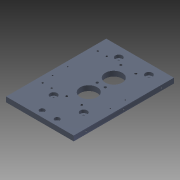
# Autodesk Inventor part: 13_0204_028
Saved by Autodesk Inventor 2012 SP1 (Build 160190100, 190)
## iProperties
Created: 2013-03-27
Part Number: 13_0204_028
Material: Default
Document SubType Name: Modeling
Designer: vogel
Density: 1 g/cm^3
Author: vogel
Autodesk Inventor part; units mm, degrees
ref_plane "YZ Plane" through (0, 0, 0) normal (1, 0, 0) x (0, 1, 0)
ref_plane "XZ Plane" through (0, 0, 0) normal (0, 1, 0) x (-1, 0, 0)
sketch "Skizze1" plane through (0, 0, 0) normal (0, 0, 1) x (1, 0, 0)
  line L0 (-60, 110) -> (60, 110)
  line L1 (60, 110) -> (60, -50)
  line L2 (60, -50) -> (-60, -50)
  line L3 (-60, -50) -> (-60, 110)
  line L4 (-1104, 0) -> (254, 0) projected
  line L5 (0, -83) -> (0, 148) projected
  circle A0 centre (-30, 0) radius 2.7
  circle A1 centre (30, 0) radius 2.7
  line L6 (-910, 115) -> (-40, 115) projected
  point P0 (0, 0)
  dimension "d0" = 110
  dimension "d1" = 120
  dimension "d2" = 60
  dimension "d3" = 5.4
  dimension "d7" = 50
  constraints: 8 end point, 2 centre point, 2 coincident, 2 parallel, 2 point on line, 1 equal radius, 1 horizontal, 1 perpendicular, 1 symmetric about line, 1 other
  measures "d0" distance between parallel lines of L0 L4
  measures "d1" distance of L0.start L0.end
  measures "d2" distance of point (30, 0) point (-30, 0)
  measures "d3" diameter of A0
  measures "d7" distance between parallel lines of L2 L4
extrude "Extrusion1" add sketch "Skizze1" along normal blind 10 contours L0 L5 L4 A0 L3 | L0 L1 L4 A1 L5 | L4 A0 L5 L2 L3 | L4 A1 L1 L2 L5
sketch "Skizze2" plane through (0, 0, 10) normal (0, 0, 1) x (1, 0, 0)
  line L0 (-60, 110) -> (60, 110) projected
  line L1 (0, -82) -> (0, 142) projected
  point P0 (0, 0)
  point P1 (0, 90)
  point P2 (0, 40)
  dimension "d17" = 20
  dimension "d18" = 50
  constraints: 2 point on line
  measures "d17" distance from line of L0 point (0, 90)
  measures "d18" distance of point (0, 90) point (0, 40)
hole "Bohrung2" at (0, 90, 10) at (0, 40, 10) direction (0, 0, -1) diameter 34 end through all
sketch "Skizze5" plane through (0, 0, 10) normal (0, 0, 1) x (1, 0, 0)
  circle A0 centre (30, 0) radius 2.7 projected
  circle A1 centre (-30, 0) radius 2.7 projected
  circle A2 centre (-30, 0) radius 7
  circle A3 centre (30, 0) radius 7
  point P0 (0, 0)
  dimension "d33" = 14
  constraints: 2 centre point, 2 coincident, 1 equal radius
  measures "d33" diameter of A2
extrude "Extrusion2" cut sketch "Skizze5" against normal blind 6
sketch "Skizze6" plane through (-60, 110, 0) normal (0, 1, 0) x (1, 0, 0)
  line L0 (0, -10) -> (120, -10) projected
  line L1 (120, 0) -> (120, -10) projected
  line L2 (0, 0) -> (120, 0) projected
  line L3 (0, 0) -> (0, -10) projected
  point P0 (60, 0)
extrude "Extrusion3" add sketch "Skizze6" along normal blind 40
pattern_linear "Rechteckige Anordnung1" count 2 spacing 130 along (0, 1, 0) of "Extrusion2"
sketch "Skizze8" plane through (0, 0, 10) normal (0, 0, 1) x (1, 0, 0)
  circle A0 centre (30, 130) radius 7 projected
  circle A1 centre (-30, 130) radius 7 projected
  point P0 (0, 0)
  constraints: 2 coincident
hole "Bohrung4" at (-30, 130, 10) at (30, 130, 10) direction (0, 0, -1) diameter 5.4 end through all
sketch "Skizze9" plane through (-60, -50, 0) normal (-1, 0, 0) x (0, 0, 1)
  line L0 (10, 0) -> (10, 200) projected
  line L1 (10, 200) -> (0, 200) projected
  line L2 (0, 0) -> (0, 200) projected
  line L3 (0, 0) -> (10, 0) projected
  point P0 (0, 50)
extrude "Extrusion4" add sketch "Skizze9" along normal blind 15
sketch "Skizze10" plane through (0, 0, 10) normal (0, 0, 1) x (1, 0, 0)
  line L0 (60, 150) -> (-75, 150) projected
  line L1 (-75, 150) -> (-75, -50) projected
  line L2 (60, -50) -> (-75, -50) projected
  line L3 (-75, 120) -> (-28.668, 120)
  line L4 (-53, 93.8234) -> (-53, 98.8806)
  line L5 (60, 150) -> (60, -50) projected
  line L6 (-75, 10) -> (-27.5048, 10)
  point P0 (0, 0)
  point P1 (-62, 120)
  point P2 (-44, 120)
  point P3 (-62, 10)
  point P4 (-44, 10)
  dimension "d50" = 30
  dimension "d51" = 22
  dimension "d52" = 18
  dimension "d60" = 140
  dimension "d61" = 18
  constraints: 6 end point, 6 point on line, 2 perpendicular, 2 symmetric about line, 1 parallel
  measures "d50" distance between parallel lines of L0 L3
  measures "d51" distance between parallel lines of L1 L4
  measures "d52" distance of point (-44, 120) point (-62, 120)
  measures "d60" distance between parallel lines of L0 L6
  measures "d61" distance of point (-44, 10) point (-62, 10)
hole "Bohrung6" at (-62, 120, 10) at (-44, 120, 10) at (-62, 10, 10) at (-44, 10, 10) direction (0, 0, -1) diameter 3.242 end through all thread size "M4x0.7" class "6H" standard "ISO Metric profile"
sketch "Skizze11" plane through (0, 0, 10) normal (0, 0, 1) x (1, 0, 0)
  circle A0 centre (7.5, -46) radius 1.621 projected
  circle A1 centre (7.5, -30) radius 1.621 projected
  circle A2 centre (-7.5, -30) radius 1.621 projected
  circle A3 centre (-7.5, -46) radius 1.621 projected
  line L0 (-25, -26) -> (25, -26) projected
  line L1 (-25, -50) -> (-25, -26) projected
  line L2 (25, -50) -> (-25, -50) projected
  line L3 (25, -26) -> (25, -50) projected
  line L4 (-25, -38) -> (25, -38)
  line L5 (-102, 0) -> (87, 0) projected
  line L6 (0, -90) -> (0, 190) projected
  circle A4 centre (15, -38) radius 2.067 projected
  circle A5 centre (-15, -38) radius 2.067 projected
  point P0 (0, 0)
  point P1 (-15, -38)
  point P2 (15, -38)
  dimension "d69" = 30
  constraints: 2 end point, 2 midpoint, 2 point on line, 1 symmetric about line
  measures "d69" distance of point (15, -38) point (-15, -38)
hole "Bohrung7" at (-15, -38, 10) at (15, -38, 10) direction (0, 0, -1) diameter 5.5 end through all counterbore diameter 10 counterbore depth 5.4
sketch "Skizze12" plane through (60, -50, 10) normal (1, 0, 0) x (0, 0, -1)
  line L0 (0, 200) -> (0, 0) projected
  line L1 (10, 0) -> (0, 0) projected
  line L2 (10, 200) -> (0, 200) projected
  line L3 (10, -40) -> (10, 240) projected
  line L4 (12, 50) -> (-2, 50) projected
  line L5 (0, 100) -> (10, 100)
  line L6 (5, 200) -> (5, 0)
  point P0 (10, 50)
  point P1 (5, 175)
  point P2 (5, 100)
  point P3 (5, 25)
  dimension "d77" = 25
  dimension "d78" = 25
  constraints: 5 midpoint, 4 end point, 2 point on line, 1 perpendicular
  measures "d77" distance of L6.start point (5, 175)
  measures "d78" distance from line of point (5, 25) L1
hole "Bohrung8" at (60, 125, 5) at (60, 50, 5) at (60, -25, 5) direction (-1, 0, 0) diameter 2.459 depth 10 tip angle 118 thread size "M3x0.5" class "6H" standard "ISO Metric profile"
ref_plane "Arbeitsebene1" through (-7.5, -50, 10) normal (1, 0, 0) x (0, 0, -1)
mirror "Spiegeln1" about plane through (-7.5, -50, 10) normal (1, 0, 0) of "Bohrung8"
hole "Bohrung9" at (8, 65, 10) at (-8, 65, 10) direction (0, 0, -1) diameter 5 end through all
sketch "Skizze13" plane through (0, 0, 10) normal (0, 0, 1) x (1, 0, 0)
  circle A0 centre (-15, 119) radius 2.75 projected
  circle A1 centre (15, 119) radius 2.75 projected
  circle A2 centre (15, 11) radius 2.75 projected
  circle A3 centre (-15, 11) radius 2.75 projected
  point P0 (0, 0)
  constraints: 4 coincident
hole "Bohrung10" at (-15, 11, 10) at (15, 11, 10) at (15, 119, 10) at (-15, 119, 10) direction (0, 0, -1) diameter 4.134 end through all thread size "M5x0.8" class "6H" standard "ISO Metric profile"
sketch "Skizze14" plane through (0, 0, 10) normal (0, 0, 1) x (1, 0, 0)
  line L0 (60, 150) -> (60, -50) projected
  line L1 (60, 150) -> (-75, 150) projected
  line L2 (-75, 150) -> (-75, -50) projected
  line L3 (60, -50) -> (-75, -50) projected
  line L4 (50, 150) -> (50, -50)
  line L5 (-65, 150) -> (-65, -50)
  point P0 (0, 0)
  point P1 (50, 63)
  point P2 (50, 33)
  point P3 (-65, 63)
  point P4 (-65, 33)
  dimension "d101" = 10
  dimension "d102" = 87
  dimension "d103" = 30
  dimension "d104" = 10
  constraints: 8 point on line, 4 end point, 2 horizontal alignment, 2 perpendicular
  measures "d101" distance between parallel lines of L4 L0
  measures "d102" distance from line of L1 point (50, 63)
  measures "d103" distance of point (50, 33) point (50, 63)
  measures "d104" distance between parallel lines of L2 L5
hole "Bohrung11" at (50, 63, 10) at (50, 33, 10) at (-65, 63, 10) at (-65, 33, 10) direction (0, 0, -1) diameter 2.459 end through all thread size "M3x0.5" class "6H" standard "ISO Metric profile"
